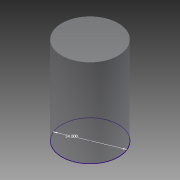
# Autodesk Inventor part: Playing Configuration Constraint
Saved by Autodesk Inventor 2013 (Build 170138000, 138)
## iProperties
Created: 2013-01-06
Part Number: Playing Configuration Constraint
Material: Generic
Document SubType Name: Modeling
Designer: Moses
Surface Area: 121488 cm^2
Density: 1 g/cm^3
Author: Moses
Autodesk Inventor part; units mm, degrees
ref_plane "XZ Plane" through (0, 0, 0) normal (0, 1, 0) x (-1, 0, 0)
ref_plane "XY Plane" through (0, 0, 0) normal (0, 0, 1) x (1, 0, 0)
sketch "Sketch1" plane through (0, 0, 0) normal (0, 1, 0) x (-1, 0, 0)
  circle A0 centre (0, 0) radius 685.8
  dimension "d0" = 1371.6
  constraints: 1 centre point, 1 coincident
  measures "d0" diameter of A0
extrude "Extrusion1" add sketch "Sketch1" along normal blind 2133.6
body "Solid1"
